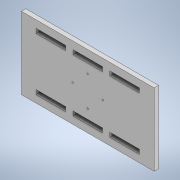
# Autodesk Inventor part: Part1
Saved by Autodesk Inventor 2022 (Build 260153000, 153)
## iProperties
Created: 2021-10-21
Part Number: Part1
Material: Generic
Document SubType Name: Modeling
Designer: Administrador
Density: 1 g/cm^3
Appearance: Default
Author: Administrador
Autodesk Inventor part; units mm, degrees
ref_plane "YZ Plane" through (0, 0, 0) normal (1, 0, 0) x (0, 1, 0)
ref_plane "XZ Plane" through (0, 0, 0) normal (0, 1, 0) x (-1, 0, 0)
ref_plane "XY Plane" through (0, 0, 0) normal (0, 0, 1) x (1, 0, 0)
sketch "Sketch1" plane through (0, 0, 0) normal (0, 0, 1) x (1, 0, 0)
  line L0 (-45, 24.5) -> (45, 24.5)
  line L1 (45, 24.5) -> (45, -24.5)
  line L2 (45, -24.5) -> (-45, -24.5)
  line L3 (-45, -24.5) -> (-45, 24.5)
  line L4 (-45, 24.5) -> (-45, 19.5)
  line L5 (-35, 19.5) -> (-15, 19.5)
  line L6 (-15, 19.5) -> (-15, 16.5)
  line L7 (-15, 16.5) -> (-35, 16.5)
  line L8 (-35, 16.5) -> (-35, 19.5)
  line L9 (-10, 19.5) -> (10, 19.5)
  line L10 (10, 19.5) -> (10, 16.5)
  line L11 (10, 16.5) -> (-10, 16.5)
  line L12 (-10, 16.5) -> (-10, 19.5)
  line L13 (10, 16.5) -> (10, 19.5)
  line L14 (-45, 0) -> (-35, 0) construction
  line L15 (-35, -19.5) -> (-15, -19.5)
  line L16 (-15, -19.5) -> (-15, -16.5)
  line L17 (-15, -16.5) -> (-35, -16.5)
  line L18 (-35, -16.5) -> (-35, -19.5)
  line L19 (-10, -19.5) -> (10, -19.5)
  line L20 (10, -19.5) -> (10, -16.5)
  line L21 (10, -16.5) -> (-10, -16.5)
  line L22 (-10, -16.5) -> (-10, -19.5)
  line L23 (10, -16.5) -> (10, -19.5)
  line L24 (15, 19.5) -> (35, 19.5)
  line L25 (35, 19.5) -> (35, 16.5)
  line L26 (35, 16.5) -> (15, 16.5)
  line L27 (15, 16.5) -> (15, 19.5)
  line L28 (15, -19.5) -> (35, -19.5)
  line L29 (35, -19.5) -> (35, -16.5)
  line L30 (35, -16.5) -> (15, -16.5)
  line L31 (15, -16.5) -> (15, -19.5)
  circle A0 centre (0, 0) radius 10.25
  circle A1 centre (-10.25, 0) radius 0.5
  circle A2 centre (10.25, 0) radius 0.5
  circle A3 centre (0, 10.25) radius 0.5
  circle A4 centre (0, -10.25) radius 0.5
  dimension "d3" = 49
  dimension "d6" = 5
  dimension "d7" = 10
  dimension "d8" = 20
  dimension "d11" = 20
  dimension "d14" = 5
  dimension "d17" = 24.5
  dimension "d19" = 20
  dimension "d20" = 5
  dimension "d23" = 20.5
  dimension "d24" = 1
  dimension "d25" = 1
  dimension "d26" = 1
  dimension "d27" = 1
  constraints: 64 end point, 10 parallel, 9 symmetric about line, 6 horizontal, 5 centre point, 5 perpendicular, 4 point on circle, 1 coincident, 1 midpoint, 1 point on line
  measures "d3" distance of L0.end L1.end
  measures "d6" distance of L0.start L4.end
  measures "d7" distance of L4.end L5.start
  measures "d8" distance of L6.end L7.end
  measures "d11" distance of L10.end L11.end
  measures "d14" distance between parallel lines of L12 L6
  measures "d17" distance from line of L0 point (0, 0)
  measures "d19" distance of L25.end L26.end
  measures "d20" distance between parallel lines of L27 L10
  measures "d23" diameter of A0
  measures "d24" diameter of A1
  measures "d25" diameter of A2
  measures "d26" diameter of A3
  measures "d27" diameter of A4
extrude "Extrusion1" add sketch "Sketch1" along normal blind 3 contours L0 L1 L2 L3 | A2 A0 A4 A1 A3
body "Solid1"
